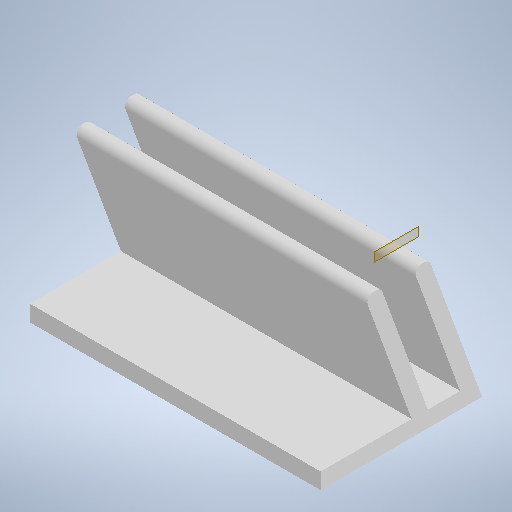
# Autodesk Inventor part: Stojan
Saved by Autodesk Inventor 2025.1 (Build 291241020, 241B)
## iProperties
Created: 2025-04-08
Part Number: Stojan
Material: Generic
Document SubType Name: Modeling
Designer: ondre
Density: 1 g/cm^3
Appearance: Default
Author: ondre
Autodesk Inventor part; units mm, degrees
ref_plane "YZ Plane" through (0, 0, 0) normal (1, 0, 0) x (0, 1, 0)
ref_plane "XZ Plane" through (0, 0, 0) normal (0, 1, 0) x (-1, 0, 0)
ref_plane "XY Plane" through (0, 0, 0) normal (0, 0, 1) x (1, 0, 0)
ref_plane "Work Plane5" through (200, 0, -20) normal (-1, 0, 0) x (0, 0, 1)
sketch "Sketch7" plane through (200, 0, -20) normal (-1, 0, 0) x (0, 0, 1)
  line L0 (0, 0) -> (10, 0) construction
  line L1 (0, 0) -> (31.7994, 87.3681)
  line L2 (35.5582, 90) -> (37.0447, 90)
  line L3 (40.8035, 84.6319) -> (13.6397, 10)
  line L4 (13.6397, 10) -> (33.6397, 10)
  line L5 (33.6397, 10) -> (61.7994, 87.3681)
  line L6 (65.5582, 90) -> (67.0447, 90)
  line L7 (70.8035, 84.6319) -> (43.6397, 10)
  line L8 (0, 0) -> (40, 0)
  line L9 (0, 0) -> (40, 0) construction
  line L10 (100, 0) -> (100, 10)
  line L11 (43.6397, 10) -> (100, 10)
  line L12 (100, 0) -> (40, 0)
  arc A0 (65.5582, 90) -> (61.7994, 87.3681) centre (65.5582, 86) ccw
  arc A1 (70.8035, 84.6319) -> (67.0447, 90) centre (67.0447, 86) ccw
  arc A2 (35.5582, 90) -> (31.7994, 87.3681) centre (35.5582, 86) ccw
  arc A3 (40.8035, 84.6319) -> (37.0447, 90) centre (37.0447, 86) ccw
  point P0 (20, 0)
  point P1 (62.7573, 90)
  point P2 (40, 0)
  dimension "d42" = 4
  constraints: 26 end point, 8 point on circle, 8 tangent, 4 centre point, 4 horizontal, 3 equal radius, 3 point on line, 2 collinear, 1 parallel
  measures "d42" radius of A0
extrude "Extrusion4" add sketch "Sketch7" along normal blind 180
body "Solid2"
